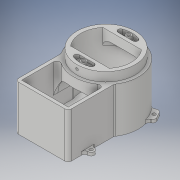
# Autodesk Inventor part: table
Saved by Autodesk Inventor 2018 (Build 220112000, 112)
## iProperties
Created: 2018-04-17
Part Number: table
Material: Generic
Document SubType Name: Modeling
Designer: Cole Tucker
Density: 1 g/cm^3
Appearance: Default
Author: Cole Tucker
Autodesk Inventor part; units mm, degrees
ref_plane "YZ Plane" through (0, 0, 0) normal (1, 0, 0) x (0, 1, 0)
ref_plane "XZ Plane" through (0, 0, 0) normal (0, 1, 0) x (-1, 0, 0)
ref_plane "XY Plane" through (0, 0, 0) normal (0, 0, 1) x (1, 0, 0)
sketch "Sketch1" plane through (0, 0, 0) normal (0, 1, 0) x (-1, 0, 0)
  circle A0 centre (0, 0) radius 24.765
  circle A1 centre (0, 0) radius 28.575
  dimension "d0" = 49.53
  dimension "d1" = 57.15
  constraints: 2 centre point, 2 coincident
  measures "d0" diameter of A0
  measures "d1" diameter of A1
extrude "Extrusion1" add sketch "Sketch1" along normal blind 53.34
sketch "Sketch2" plane through (0, 0, 0) normal (0, -1, 0) x (1, 0, 0)
  circle A0 centre (0, 0) radius 31.75
  circle A1 centre (0, 0) radius 24.765 projected
  circle A2 centre (0, 0) radius 28.575 projected
  circle A3 centre (0, 0) radius 28.575
  dimension "d4" = 63.5
  constraints: 2 centre point, 2 coincident
  measures "d4" diameter of A0
extrude "Extrusion2" add sketch "Sketch2" against normal blind 44.45 contours A0
sketch "Sketch3" plane through (0, 0, 0) normal (0, -1, 0) x (1, 0, 0)
  circle A0 centre (0, 0) radius 24.765 projected
  line L0 (0, 24.765) -> (6.35, 24.765)
  line L1 (6.35, 24.765) -> (6.35, 37.465)
  line L2 (6.35, 37.465) -> (-6.35, 37.465)
  line L3 (-6.35, 37.465) -> (-6.35, 24.765)
  line L4 (-6.35, 24.765) -> (0, 24.765)
  dimension "d7" = 6.35
  dimension "d8" = 12.7
  dimension "d9" = 12.7
  constraints: 10 end point, 3 horizontal, 3 perpendicular, 1 collinear, 1 point on line, 1 vertical alignment, 1 other
  measures "d7" distance of L0.start L0.end
  measures "d8" distance of L0.end L1.end
  measures "d9" distance of L1.end L2.end
extrude "Extrusion3" add sketch "Sketch3" against normal blind 3.175 contours L4 L3 L2 L1 L0
pattern_circular "Circular Pattern3" count 3 over 360 about axis through (0, 0, 0) along (0, 1, 0) of "Extrusion3"
sketch "Sketch5" plane through (0, 3.175, 0) normal (0, 1, 0) x (1, 0, 0)
  line L0 (6.35, -37.465) -> (-6.35, -37.465) projected
  line L1 (0, -37.465) -> (0, -31.75)
  circle A0 centre (0, 0) radius 31.75 projected
  point P0 (0, -34.6075)
  constraints: 2 end point, 2 midpoint, 1 vertical, 1 vertical alignment, 1 other
hole "Hole2" at (0, 3.175, 34.6075) direction (0, -1, 0) diameter 3.175 end through all
pattern_circular "Circular Pattern4" count 3 over 360 about axis through (0, 0, 0) along (0, 1, 0) of "Hole2"
sketch "Sketch6" plane through (-6.35, 0, 37.465) normal (0, 0, 1) x (1, 0, 0)
  line L0 (12.7, 3.175) -> (0, 3.175) projected
  line L1 (6.35, 3.175) -> (6.35, 34.925)
  line L2 (6.35, 34.925) -> (-16.51, 34.925)
  line L3 (-16.51, 34.925) -> (-16.51, 3.175)
  line L4 (-16.51, 3.175) -> (6.35, 3.175)
  line L5 (6.35, 3.175) -> (29.21, 3.175)
  line L6 (29.21, 3.175) -> (29.21, 34.925)
  line L7 (29.21, 34.925) -> (6.35, 34.925)
  point P0 (6.35, 0)
  dimension "d38" = 31.75
  dimension "d39" = 22.86
  dimension "d40" = 22.86
  constraints: 14 end point, 4 perpendicular, 2 point on line, 1 collinear, 1 midpoint, 1 vertical
  measures "d38" distance of L1.start L1.end
  measures "d39" distance of L1.end L2.end
  measures "d40" distance of L1.start L5.end
extrude "Extrusion4" cut sketch "Sketch6" against normal blind 38.1
sketch "Sketch7" plane through (0, 3.175, 0) normal (0, 1, 0) x (1, 0, 0)
  circle A0 centre (0, 0) radius 24.765
  constraints: 1 centre point, 1 coincident
extrude "Extrusion5" add sketch "Sketch7" against normal blind 3.175
sketch "Sketch8" plane through (0, 3.175, 0) normal (0, 1, 0) x (1, 0, 0)
  line L0 (-22.86, -22.0337) -> (-22.86, -9.525) projected
  line L1 (-22.86, -22.0337) -> (22.86, -22.0337)
  line L2 (22.86, -22.0337) -> (22.86, -60.1337)
  line L3 (22.86, -60.1337) -> (-22.86, -60.1337)
  line L4 (-22.86, -60.1337) -> (-22.86, -22.0337)
  point P0 (0, 0)
  dimension "d45" = 38.1
  constraints: 8 end point, 2 parallel, 1 horizontal, 1 perpendicular
  measures "d45" distance of L1.end L2.end
extrude "Extrusion6" add sketch "Sketch8" against normal blind 3.175
sketch "Sketch9" plane through (0, 0, 0) normal (0, -1, 0) x (1, 0, 0)
  line L0 (-22.86, 60.1337) -> (-22.86, 22.0337) projected
  line L1 (-22.86, 60.1337) -> (-26.035, 60.1337)
  line L2 (-26.035, 60.1337) -> (-26.035, 63.3087)
  line L3 (-26.035, 63.3087) -> (-22.86, 63.3087)
  line L4 (-22.86, 63.3087) -> (-22.86, 60.1337)
  line L5 (22.86, 22.0337) -> (22.86, 60.1337) projected
  line L6 (22.86, 60.1337) -> (26.035, 60.1337)
  line L7 (26.035, 60.1337) -> (26.035, 63.3087)
  line L8 (26.035, 63.3087) -> (22.86, 63.3087)
  line L9 (22.86, 63.3087) -> (22.86, 60.1337)
  line L10 (26.035, 60.1337) -> (26.035, 18.1725)
  arc A0 (30.1158, -10.055) -> (22.86, 22.0337) centre (0, 0) ccw projected
  line L11 (-22.86, 63.3087) -> (22.86, 63.3087)
  line L12 (-26.035, 60.1337) -> (-26.035, 18.1725)
  arc A1 (-22.86, 22.0337) -> (-30.1158, -10.055) centre (0, 0) ccw projected
  dimension "d48" = 3.175
  dimension "d49" = 3.175
  dimension "d50" = 3.175
  dimension "d51" = 3.175
  constraints: 22 end point, 4 parallel, 3 perpendicular, 2 horizontal, 2 point on circle, 1 vertical
  measures "d48" distance of L2.end L3.end
  measures "d49" distance of L1.end L2.end
  measures "d50" distance of L8.end L7.end
  measures "d51" distance of L7.end L6.end
extrude "Extrusion7" add sketch "Sketch9" against normal blind 44.45
sketch "Sketch10" plane through (0, 0, 0) normal (0, -1, 0) x (1, 0, 0)
  line L0 (-22.86, 60.1337) -> (-22.86, 63.3087) projected
  line L1 (22.86, 60.1337) -> (-22.86, 60.1337) projected
  line L2 (-22.86, 63.3087) -> (22.86, 63.3087)
  line L3 (22.86, 63.3087) -> (22.86, 60.1337)
  line L4 (22.86, 60.1337) -> (-22.86, 60.1337)
  line L5 (-22.86, 60.1337) -> (-22.86, 63.3087)
  point P0 (0, 0)
  constraints: 8 end point, 2 parallel, 1 horizontal, 1 perpendicular
extrude "Extrusion8" add sketch "Sketch10" against normal blind 44.45
sketch "Sketch11" plane through (0, 0, 0) normal (0, -1, 0) x (1, 0, 0)
  line L0 (-26.035, 18.1725) -> (-26.035, 63.3087) projected
  line L1 (-26.035, 40.7406) -> (-32.385, 40.7406)
  line L2 (-32.385, 40.7406) -> (-32.385, 47.0906)
  line L3 (-32.385, 47.0906) -> (-26.035, 47.0906)
  line L4 (-26.035, 47.0906) -> (-26.035, 40.7406)
  point P0 (0, 0)
  dimension "d56" = 6.35
  dimension "d57" = 6.35
  constraints: 8 end point, 2 parallel, 1 horizontal, 1 midpoint, 1 perpendicular
  measures "d56" distance of L2.end L3.end
  measures "d57" distance of L1.end L2.end
extrude "Extrusion9" add sketch "Sketch11" against normal blind 3.175
sketch "Sketch12" plane through (0, 0, 0) normal (0, -1, 0) x (1, 0, 0)
  line L0 (-26.035, 40.7406) -> (-32.385, 40.7406) projected
  line L1 (-29.21, 40.7406) -> (-29.21, 47.0906)
  line L2 (-32.385, 47.0906) -> (-26.035, 47.0906) projected
  point P0 (0, 0)
  point P1 (-29.21, 43.9156)
  constraints: 3 midpoint, 2 end point
hole "Hole3" at (-29.21, 0, 43.9156) direction (0, 1, 0) diameter 3.175 end through all
ref_plane "Work Plane1" through (0, 0, 63.3087) normal (-1, 0, 0) x (0, 0, 1)
mirror "Mirror1" about plane through (0, 0, 63.3087) normal (-1, 0, 0) of "Extrusion9", "Hole3"
fillet "Fillet1" radius 3.175 4 edges at (26.035, 1.5875, 47.0906) (26.035, 1.5875, 40.7406) (32.385, 1.5875, 40.7406) (32.385, 1.5875, 47.0906)
fillet "Fillet2" radius 3.175 4 edges at (-26.035, 1.5875, 40.7406) (-32.385, 1.5875, 40.7406) (-32.385, 1.5875, 47.0906) (-26.035, 1.5875, 47.0906)
fillet "Fillet3" radius 3.175 8 edges at (-35.6206, 1.5875, -13.2332) (-30.1158, 1.5875, -10.055) (-29.2706, 1.5875, -24.2318) (-23.7658, 1.5875, -21.0535) (30.1158, 1.5875, -10.055) (35.6206, 1.5875, -13.2332) (29.2706, 1.5875, -24.2318) (23.7658, 1.5875, -21.0535)
fillet "Fillet4" radius 3.175 2 edges at (-22.86, 19.05, 9.525) (22.86, 19.05, 9.525)
fillet "Fillet5" radius 3.175 2 edges at (-26.035, 22.225, 18.1725) (26.035, 22.225, 18.1725)
fillet "Fillet6" radius 3.175 2 edges at (26.035, 22.225, 63.3087) (-26.035, 22.225, 63.3087)
fillet "Fillet7" radius 3.175 2 edges at (-22.86, 39.6875, 22.0337) (22.86, 39.6875, 22.0337)
fillet "Fillet8" radius 19.05 6 edges at (22.9146, 34.925, 9.5539) (22.86, 34.925, 25.4413) (22.86, 34.925, 16.0869) (-22.9146, 34.925, 9.5539) (-22.86, 34.925, 25.4413) (-22.86, 34.925, 16.0869)
sketch "Sketch13" plane through (0, 53.34, 0) normal (0, 1, 0) x (1, 0, 0)
  circle A0 centre (0, 0) radius 24.765 projected
  line L0 (0, 24.765) -> (-19.05, 24.765)
  line L1 (-19.05, 24.765) -> (-19.05, 15.8241)
  line L2 (-19.05, 15.8241) -> (19.05, 15.8241)
  arc A1 (-3.81, -24.4702) -> (3.81, -24.4702) centre (0, 0) ccw projected
  line L3 (0, -24.765) -> (-19.05, -24.765)
  line L4 (-19.05, -24.765) -> (-19.05, -15.8241)
  line L5 (-19.05, -15.8241) -> (19.05, -15.8241)
  dimension "d79" = 19.05
  dimension "d80" = 19.05
  constraints: 12 end point, 4 horizontal, 4 perpendicular, 1 point on circle, 1 tangent, 6 other
  measures "d79" distance of L0.start L0.end
  measures "d80" distance of L3.start L3.end
extrude "Extrusion10" add sketch "Sketch13" against normal blind 8.89 contours L2 A0 | A0 L5
fillet "Fillet9" radius 6.35 2 edges at (0, 44.45, 24.765) (0, 44.45, -24.765)
sketch "Sketch14" plane through (0, 53.34, 0) normal (0, 1, 0) x (1, 0, 0)
  line L0 (-9.4186, -15.8241) -> (9.4186, -15.8241) construction
  line L1 (0, -15.8241) -> (0, -28.575) construction
  circle A0 centre (0, 0) radius 28.575 construction
  line L2 (0, 28.575) -> (0, 15.8241) construction
  line L3 (9.4186, 15.8241) -> (-9.4186, 15.8241) construction
  point P0 (0, -22.1996)
  point P1 (0, 22.1996)
  constraints: 4 end point, 4 midpoint, 2 point on circle, 1 vertical
hole "Hole4" at (0, 53.34, 22.1996) at (0, 53.34, -22.1996) direction (0, -1, 0) diameter 3.175 depth 25.4 tip angle 118
sketch "Sketch15" plane through (-26.035, 0, 37.5656) normal (-1, 0, 0) x (0, 0, 1)
  line L0 (22.5681, 3.175) -> (-27.4255, 3.175) construction
  line L1 (-2.4287, 3.175) -> (-2.4287, 9.525) construction
  point P0 (-37.5656, 0)
  dimension "d95" = 6.35
  constraints: 2 end point, 1 coincident, 1 midpoint, 1 vertical
  measures "d95" distance of L1.start L1.end
hole "Hole5" at (-26.035, 9.525, 35.1369) direction (1, 0, 0) diameter 6.35 depth 25.4 tip angle 118
sketch "Sketch16" plane through (0, 53.34, 0) normal (0, 1, 0) x (1, 0, 0)
  line L0 (19.05, -15.8241) -> (-19.05, -15.8241) construction
  line L1 (0, -15.8241) -> (0, -18.9991) construction
  circle A0 centre (0, 0) radius 28.575 construction
  line L2 (0, -28.575) -> (0, -25.4) construction
  line L3 (0, -18.9991) -> (15.8852, -18.9991)
  arc A1 (-19.05, -15.8241) -> (19.05, -15.8241) centre (0, 0) ccw projected
  line L4 (0, -18.9991) -> (-15.8852, -18.9991)
  arc A2 (-15.8852, -18.9991) -> (15.8852, -18.9991) centre (0, -2.4883) ccw
  circle A3 centre (0, -22.1996) radius 1.5875 projected
  circle A4 centre (0, -22.1996) radius 2.54
  dimension "d103" = 3.175
  dimension "d104" = 3.175
  dimension "d105" = 5.08
  constraints: 8 end point, 5 point on circle, 2 centre point, 2 vertical, 1 coincident, 1 horizontal, 1 midpoint, 1 point on line, 1 vertical alignment, 1 other
  measures "d103" distance of L1.start L1.end
  measures "d104" distance of L2.start L2.end
  measures "d105" diameter of A4
extrude "Extrusion11" cut sketch "Sketch16" against normal blind 5.08 contours L3 A1 L4 | A2 A1
ref_plane "Work Plane2" through (0, 0, 28.575) normal (0, 0, 1) x (1, 0, 0)
sketch "Sketch17" plane through (0, 0, 28.575) normal (0, 0, 1) x (1, 0, 0)
  line L0 (-15.8852, 48.26) -> (15.8852, 48.26) construction
  line L1 (0, 48.26) -> (0, 49.53) construction
  point P0 (0, 0)
  dimension "d108" = 1.27
  constraints: 2 end point, 1 coincident, 1 midpoint, 1 vertical
  measures "d108" distance of L1.start L1.end
hole "Hole6" at (0, 49.53, 28.575) direction (0, 0, -1) diameter 2.54 depth 3.81
pattern_circular "Circular Pattern5" count 2 over 360 about axis through (0, 0, 0) along (0, 1, 0) of "Extrusion11", "Hole6"
fillet "Fillet10" radius 2.54 3 edges at (0, 48.26, 18.9991) (15.8852, 50.8, 18.9991) (-15.8852, 50.8, 18.9991)
pattern_circular "Circular Pattern6" count 2 over 360 about axis through (0, 0, 0) along (0, 1, 0) of "Fillet10"
body "Solid1"
